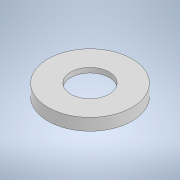
# Autodesk Inventor part: Корпус сальника
Saved by Autodesk Inventor 2021 (Build 250183000, 183)
## iProperties
Created: 2020-11-05
Part Number: Корпус сальника
Material: Типовые
Document SubType Name: Modeling
Designer: Тимоха
Density: 1 g/cm^3
Appearance: По умолчанию
Author: Тимоха
Autodesk Inventor part; units mm, degrees
ref_plane "YZ Plane" through (0, 0, 0) normal (1, 0, 0) x (0, 1, 0)
ref_plane "XZ Plane" through (0, 0, 0) normal (0, 1, 0) x (-1, 0, 0)
ref_plane "XY Plane" through (0, 0, 0) normal (0, 0, 1) x (1, 0, 0)
sketch "Эскиз1" plane through (0, 0, 0) normal (0, 0, 1) x (1, 0, 0)
  line L0 (0, 0) -> (0, 20)
  line L1 (0, 20) -> (70, 20)
  line L2 (70, 20) -> (70, 0)
  line L3 (70, 0) -> (50, 0)
  line L4 (50, 0) -> (50, 12)
  line L5 (50, 12) -> (0, 12)
  line L6 (0, 20) -> (32, 20)
  line L7 (32, 20) -> (32, 12)
  line L8 (32, 12) -> (32, 20)
  line L9 (32, 20) -> (70, 20)
  dimension "d1" = 70
  dimension "d2" = 20
  dimension "d3" = 12
  dimension "d4" = 32
  dimension "d6" = 8
  constraints: 20 end point, 7 perpendicular, 5 point on line, 1 vertical
  measures "d1" distance of L0.end L1.end
  measures "d2" distance of L2.end L3.end
  measures "d3" distance of L3.end L4.end
  measures "d4" distance of L0.end L6.end
  measures "d6" distance of L7.end L8.end
revolve "Вращение1" add sketch "Эскиз1" angle 360 about axis through (0, 0, 0) along (0, 1, 0) contours L7 L1 L2 L3 L4 L5
